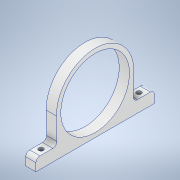
# Autodesk Inventor part: Soporte_Motor_Encoder
Saved by Autodesk Inventor 2022.1 (Build 261234000, 234)
## iProperties
Created: 2021-10-03
Part Number: Soporte_Motor_Encoder
Material: Aluminio 6061
Document SubType Name: Modeling
Designer: seb_0
Density: 2.7 g/cm^3
Appearance: Aluminio - Plano
Author: seb_0
Autodesk Inventor part; units mm, degrees
ref_plane "YZ Plane" through (0, 0, 0) normal (1, 0, 0) x (0, 1, 0)
ref_plane "XZ Plane" through (0, 0, 0) normal (0, 1, 0) x (-1, 0, 0)
ref_plane "XY Plane" through (0, 0, 0) normal (0, 0, 1) x (1, 0, 0)
sketch "Boceto1" plane through (0, 0, 0) normal (1, 0, 0) x (0, 1, 0)
  circle A0 centre (0, 0) radius 43.5
  circle A1 centre (0, 0) radius 49
  line L0 (-49, 75) -> (-49, -75)
  line L1 (-49, 75) -> (-34, 75)
  line L2 (-49, -75) -> (-34, -75)
  line L3 (-34, -75) -> (-34, -48.445)
  line L4 (-34, -48.445) -> (-0.8094, -48.9933)
  line L5 (-34, 75) -> (-34, 48.445)
  line L6 (-34, 48.445) -> (-0.8094, 48.9933)
  point P0 (-49, 0)
  dimension "d0" = 87
  dimension "d2" = 98
  dimension "d3" = 150
  dimension "d4" = 15
  constraints: 14 end point, 3 point on circle, 3 tangent, 2 centre point, 2 coincident, 2 equal length, 2 horizontal, 1 midpoint, 1 perpendicular, 1 point on line, 1 vertical
  measures "d0" diameter of A0
  measures "d2" diameter of A1
  measures "d3" distance of L0.start L0.end
  measures "d4" distance between parallel lines of L0 L3
extrude "Extrusión1" add sketch "Boceto1" along normal blind 13
fillet "Empalme1" radius 5 4 edges at (6.5, -34, 75) (6.5, -34, -75) (6.5, -34, -48.445) (6.5, -34, 48.445)
sketch "Boceto2" plane through (0, -34, 70) normal (0, 1, -0.0000001) x (1, 0, 0)
  circle A0 centre (6.5, 8) radius 3
  circle A1 centre (6.5, 132) radius 3
  line L0 (0, 16.4717) -> (0, 0) projected
  line L1 (0, -5) -> (13, -5) projected
  line L2 (13, 145) -> (0, 145) projected
  line L3 (0, 140) -> (0, 123.5283) projected
  point P0 (0, 70)
  dimension "d8" = 6
  dimension "d9" = 6
  dimension "d10" = 6.5
  dimension "d11" = 13
  dimension "d12" = 13
  dimension "d13" = 6.5
  constraints: 2 centre point
  measures "d8" diameter of A0
  measures "d9" diameter of A1
  measures "d10" distance from line of L0 A0.centre
  measures "d11" distance from line of L1 A0.centre
  measures "d12" distance from line of L2 A1.centre
  measures "d13" distance from line of L3 A1.centre
extrude "Extrusión2" cut sketch "Boceto2" against normal through all
